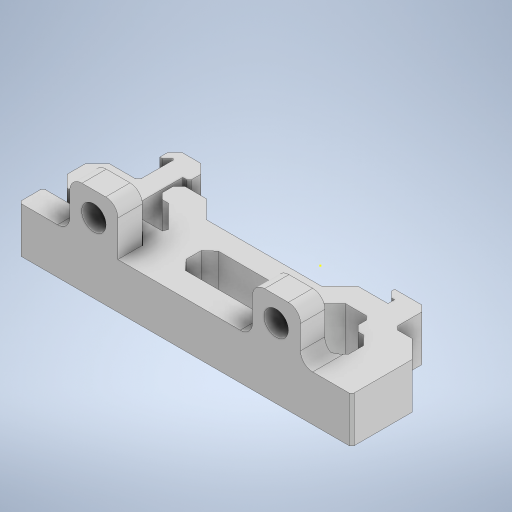
# Autodesk Inventor part: CO-1-01-lowPowerFuseMount
Saved by Autodesk Inventor 2024 (Build 280153000, 153)
## iProperties
Created: 2023-12-08
Part Number: CO-1-01-lowPowerFuseMount
Material: Generic
Document SubType Name: Modeling
Designer: t205b
Density: 1 g/cm^3
Appearance: Default
Author: t205b
Autodesk Inventor part; units mm, degrees
ref_plane "YZ Plane" through (0, 0, 0) normal (1, 0, 0) x (0, 1, 0)
ref_plane "XZ Plane" through (0, 0, 0) normal (0, 1, 0) x (-1, 0, 0)
ref_plane "XY Plane" through (0, 0, 0) normal (0, 0, 1) x (1, 0, 0)
sketch "Sketch1" plane through (0, 0, 0) normal (0, 1, 0) x (-1, 0, 0)
  point P0 (0, 0)
sketch "Sketch2" plane through (0, 0, 0) normal (0, 1, 0) x (-1, 0, 0)
  line L0 (-10.5015, 10.3489) -> (8.3899, 10.3489)
  line L1 (-25.4159, 10.3488) -> (-23.0295, 10.3488)
  line L2 (-26.8079, 11.7408) -> (-25.4159, 10.3488)
  line L3 (-28.3987, 13.3316) -> (-26.8079, 11.7408)
  line L4 (10.1121, 14.8658) -> (10.4033, 15.5686)
  line L5 (4.4127, 15.1552) -> (2.9213, 13.8428)
  line L6 (4.4127, 17.627) -> (2.9213, 19.2973)
  line L7 (25.8873, 23.2746) -> (-28.0034, 23.2746)
  line L8 (25.8893, 19.2989) -> (9.8813, 19.2989)
  line L9 (-22.433, 15.3341) -> (-20.9416, 13.8427)
  line L10 (25.8873, 23.2746) -> (26.2867, 22.8772)
  line L11 (26.2867, 22.8772) -> (26.2867, 19.6955)
  line L12 (26.2867, 19.6955) -> (25.8893, 19.2989)
  line L13 (9.8813, 19.2989) -> (11.8699, 17.3104)
  line L14 (11.8699, 17.3104) -> (24.2985, 17.3104)
  line L15 (24.2985, 17.3104) -> (26.287, 15.3218)
  line L16 (26.287, 15.3218) -> (26.287, 12.3389)
  line L17 (26.287, 12.3389) -> (24.2985, 10.3504)
  line L18 (24.2985, 10.3504) -> (20.0728, 10.3504)
  line L19 (20.0728, 10.3504) -> (19.5756, 9.8532)
  line L20 (19.5756, 9.8532) -> (19.5756, 4.6132)
  line L21 (19.5756, 4.6132) -> (19.8142, 4.3752)
  line L22 (19.8142, 4.3752) -> (20.719, 5.2815)
  line L23 (20.719, 5.2815) -> (21.1168, 5.2815)
  line L24 (21.1168, 5.2815) -> (21.1168, 3.9888)
  line L25 (21.1168, 3.9888) -> (19.9236, 2.7937)
  line L26 (19.9236, 2.7937) -> (16.8413, 2.7937)
  line L27 (16.8413, 2.7937) -> (15.3002, 4.3349)
  line L28 (15.3002, 5.9257) -> (15.3002, 4.3349)
  line L29 (15.6482, 6.2737) -> (16.3442, 6.2737)
  line L30 (10.1121, 14.8658) -> (13.8585, 11.1194)
  line L31 (13.8585, 11.1194) -> (14.8528, 11.1194)
  line L32 (14.8528, 11.1194) -> (15.847, 10.1252)
  line L33 (15.847, 10.1252) -> (15.847, 8.3603)
  line L34 (15.847, 8.3603) -> (14.8528, 7.366)
  line L35 (14.8528, 7.366) -> (11.3728, 7.366)
  line L36 (11.3728, 7.366) -> (8.3899, 10.3489)
  line L37 (-10.5015, 10.3489) -> (-13.4844, 7.366)
  line L38 (-13.4844, 7.366) -> (-18.4558, 7.366)
  line L39 (-18.4558, 7.366) -> (-18.4558, 6.2722)
  line L40 (-18.4558, 6.2722) -> (-17.9587, 6.2722)
  line L41 (-17.9587, 6.2722) -> (-16.9644, 5.2779)
  line L42 (-16.9644, 5.2779) -> (-16.9644, 4.7808)
  line L43 (-16.9644, 4.7808) -> (-21.4387, 4.7808)
  line L44 (-21.4387, 4.7808) -> (-22.433, 5.7751)
  line L45 (-22.433, 5.7751) -> (-22.433, 9.7522)
  line L46 (-22.433, 9.7522) -> (-23.0295, 10.3488)
  line L47 (-28.3987, 13.3316) -> (-28.3987, 22.8766)
  line L48 (-28.3987, 22.8766) -> (-28.0034, 23.2746)
  line L49 (-22.433, 15.3341) -> (-22.433, 17.8059)
  line L50 (-22.433, 17.8059) -> (-20.9416, 19.2973)
  line L51 (-20.9416, 19.2973) -> (2.9213, 19.2973)
  line L52 (4.4127, 17.627) -> (4.4127, 15.1552)
  line L53 (2.9213, 13.8428) -> (-11.9488, 13.8428)
  line L54 (-14.9316, 10.8599) -> (-18.4558, 10.8599)
  line L55 (-19.0524, 12.8485) -> (-20.0467, 13.8427)
  line L56 (-19.0524, 11.4565) -> (-19.0524, 12.8485)
  line L57 (-20.0467, 13.8427) -> (-20.9416, 13.8427)
  line L58 (-18.4558, 10.8599) -> (-19.0524, 11.4565)
  line L59 (-11.9488, 13.8428) -> (-14.9316, 10.8599)
  line L60 (19.3407, 12.8496) -> (19.3407, 14.8108)
  line L61 (19.3407, 14.8108) -> (23.2904, 14.8108)
  line L62 (23.2904, 14.8108) -> (23.7876, 14.3136)
  line L63 (23.7876, 14.3136) -> (23.7876, 13.3468)
  line L64 (23.7876, 13.3468) -> (23.2904, 12.8496)
  line L65 (23.2904, 12.8496) -> (19.3407, 12.8496)
  line L66 (15.6482, 6.2737) -> (15.3002, 5.9257)
  line L67 (16.3442, 15.0715) -> (16.3442, 6.2737)
  line L68 (15.847, 15.5686) -> (16.3442, 15.0715)
  line L69 (15.847, 15.5686) -> (10.4033, 15.5686)
  point P0 (0, 0)
  point P1 (-22.433, 16.57)
  dimension "d0" = 9.545
  dimension "d1" = 3.9771
  dimension "d2" = 4.4743
  dimension "d3" = 4.9714
  dimension "d4" = 3.5242
  dimension "d5" = 2.9829
  dimension "d6" = 0.9943
  dimension "d7" = 0.398
  dimension "d8" = 53.8907
  dimension "d9" = 2.4718
  dimension "d10" = 1.4914
  dimension "d11" = 1.4914
  dimension "d12" = 1.392
  dimension "d13" = 0.5966
  dimension "d14" = 23.8629
  dimension "d15" = 1.4914
  dimension "d16" = 2.4718
  dimension "d17" = 14.8701
  dimension "d18" = 2.9829
  dimension "d19" = 18.8914
  dimension "d20" = 2.9829
  dimension "d21" = 2.9829
  dimension "d22" = 3.48
  dimension "d23" = 3.7464
  dimension "d24" = 0.7028
  dimension "d25" = 5.4437
  dimension "d26" = 8.7978
  dimension "d27" = 0.4971
  dimension "d28" = 1.5909
  dimension "d29" = 0.348
  dimension "d30" = 0.696
  dimension "d31" = 1.5411
  dimension "d32" = 3.0823
  dimension "d33" = 1.1931
  dimension "d34" = 1.2927
  dimension "d35" = 0.3977
  dimension "d36" = 0.9048
  dimension "d37" = 0.2386
  dimension "d38" = 5.24
  dimension "d39" = 0.4971
  dimension "d40" = 4.2257
  dimension "d41" = 1.9886
  dimension "d42" = 2.9829
  dimension "d43" = 1.9886
  dimension "d44" = 12.4286
  dimension "d45" = 1.9886
  dimension "d46" = 16.008
  dimension "d47" = 0.3973
  dimension "d48" = 3.1817
  dimension "d49" = 2.9829
  dimension "d50" = 2.9829
  dimension "d51" = 2.9829
  dimension "d52" = 0.9943
  dimension "d53" = 0.9943
  dimension "d54" = 0.9943
  dimension "d55" = 3.7463
  dimension "d56" = 1.7649
  dimension "d57" = 0.9943
  dimension "d58" = 0.9943
  dimension "d59" = 0.4971
  dimension "d60" = 0.4971
  dimension "d61" = 0.4971
  dimension "d62" = 0.4971
  dimension "d63" = 0.4971
  constraints: 140 end point, 26 parallel, 17 perpendicular, 3 vertical, 1 horizontal, 1 midpoint
  measures "d0" distance of L47.end L3.start
  measures "d1" distance of L46.start L45.start
  measures "d2" distance of L44.start L43.start
  measures "d3" distance of L38.end L37.end
  measures "d4" distance of L54.start L54.end
  measures "d5" horizontal distance of L1.start L3.start
  measures "d6" horizontal distance of L45.start L44.start
  measures "d7" vertical distance of L7.end L47.end
  measures "d8" distance of L7.start L7.end
  measures "d9" distance of L9.start L49.end
  measures "d10" horizontal distance of L49.end L51.start
  measures "d11" horizontal distance of L9.start L57.end
  measures "d12" distance of L58.end L56.end
  measures "d13" vertical distance of L54.end L58.end
  measures "d14" distance of L51.start L6.end
  measures "d15" horizontal distance of L6.start L6.end
  measures "d16" distance of L6.start L5.start
  measures "d17" distance of L5.end L59.start
  measures "d18" horizontal distance of L59.start L54.start
  measures "d19" distance of L0.end L37.start
  measures "d20" horizontal distance of L37.end L37.start
  measures "d21" horizontal distance of L0.end L36.start
  measures "d22" distance of L36.start L35.start
  measures "d23" horizontal distance of L30.end L4.start
  measures "d24" vertical distance of L4.start L4.end
  measures "d25" distance of L4.end L68.start
  measures "d26" distance of L67.start L67.end
  measures "d27" horizontal distance of L68.start L67.start
  measures "d28" distance of L28.start L28.end
  measures "d29" horizontal distance of L28.start L29.start
  measures "d30" distance of L67.end L29.start
  measures "d31" horizontal distance of L28.end L26.end
  measures "d32" distance of L26.end L25.end
  measures "d33" horizontal distance of L25.end L24.end
  measures "d34" distance of L24.end L23.end
  measures "d35" distance of L23.end L23.start
  measures "d36" horizontal distance of L23.start L22.start
  measures "d37" horizontal distance of L22.start L20.end
  measures "d38" distance of L20.end L19.end
  measures "d39" horizontal distance of L19.end L19.start
  measures "d40" distance of L19.start L18.start
  measures "d41" horizontal distance of L16.end L18.start
  measures "d42" distance of L15.end L16.end
  measures "d43" horizontal distance of L15.start L15.end
  measures "d44" distance of L15.start L13.end
  measures "d45" horizontal distance of L13.start L13.end
  measures "d46" distance of L13.start L8.start
  measures "d47" horizontal distance of L8.start L12.start
  measures "d48" distance of L12.start L10.end
  measures "d49" horizontal distance of L37.end L37.start
  measures "d50" horizontal distance of L59.start L54.start
  measures "d51" horizontal distance of L0.end L36.start
  measures "d52" horizontal distance of L33.start L31.end
  measures "d53" horizontal distance of L33.start L31.end
  measures "d54" distance of L31.end L30.end
  measures "d55" vertical distance of L30.end L4.start
  measures "d56" distance of L33.end L33.start
  measures "d57" horizontal distance of L35.start L33.end
  measures "d58" horizontal distance of L35.start L33.end
  measures "d59" horizontal distance of L19.end L19.start
  measures "d60" horizontal distance of L63.end L65.start
  measures "d61" horizontal distance of L63.end L65.start
  measures "d62" horizontal distance of L61.end L62.end
  measures "d63" horizontal distance of L61.end L62.end
extrude "Extrusion1" add sketch "Sketch2" along normal blind 7.5
sketch "Sketch3" plane through (-25.8873, 0, 23.2746) normal (0, 0, 1) x (1, 0, 0)
  line L0 (0, 0) -> (53.8907, 0) projected
  line L1 (53.8907, 0) -> (53.8907, 7.5) projected
  line L2 (0, 7.5) -> (53.8907, 7.5) projected
  line L3 (0, 0) -> (0, 7.5) projected
  line L4 (7.9953, 7.5) -> (7.9953, 15.4)
  line L5 (7.9953, 15.4) -> (15.8953, 15.4)
  line L6 (15.8953, 15.4) -> (15.8953, 7.5)
  line L7 (37.9953, 7.5) -> (37.9953, 15.4)
  line L8 (37.9953, 15.4) -> (45.8953, 15.4)
  line L9 (45.8953, 15.4) -> (45.8953, 7.5)
  point P0 (25.8873, 0)
  dimension "d94" = 7.9
  dimension "d95" = 7.9
  dimension "d96" = 7.9
  dimension "d97" = 22.1
  dimension "d98" = 53.8907
  dimension "d99" = 7.9953
  constraints: 12 end point, 6 point on line, 3 perpendicular, 1 parallel, 1 vertical
  measures "d94" distance between parallel lines of L7 L9
  measures "d95" distance between parallel lines of L8 L2
  measures "d96" distance between parallel lines of L4 L6
  measures "d97" distance between parallel lines of L7 L6
  measures "d98" distance between parallel lines of L3 L1
  measures "d99" distance between parallel lines of L4 L3
extrude "Extrusion2" add sketch "Sketch3" against normal blind 4 contours L4 L5 L6 L2 | L2 L7 L8 L9
fillet "Fillet1" radius 2 7 edges at (-17.892, 15.4, 21.2746) (-17.892, 7.5, 21.2868) (-9.992, 15.4, 21.2746) (12.108, 15.4, 21.2746) (20.008, 15.4, 21.2746) (20.008, 7.5, 21.286) (12.108, 7.5, 21.286)
sketch "Sketch4" plane through (-25.8873, 0, 23.2746) normal (0, 0, 1) x (1, 0, 0)
  arc A0 (45.8953, 13.4) -> (43.8953, 15.4) centre (43.8953, 13.4) ccw projected
  line L0 (43.8953, 15.4) -> (39.9953, 15.4) projected
  arc A1 (39.9953, 15.4) -> (37.9953, 13.4) centre (39.9953, 13.4) ccw projected
  line L1 (37.9953, 13.4) -> (37.9953, 9.5) projected
  arc A2 (35.9953, 7.5) -> (37.9953, 9.5) centre (35.9953, 9.5) ccw projected
  line L2 (15.8953, 7.5) -> (35.9953, 7.5) projected
  line L3 (15.8953, 7.5) -> (15.8953, 13.4) projected
  arc A3 (15.8953, 13.4) -> (13.8953, 15.4) centre (13.8953, 13.4) ccw projected
  line L4 (13.8953, 15.4) -> (9.9953, 15.4) projected
  arc A4 (9.9953, 15.4) -> (7.9953, 13.4) centre (9.9953, 13.4) ccw projected
  line L5 (7.9953, 13.4) -> (7.9953, 9.5) projected
  arc A5 (5.9953, 7.5) -> (7.9953, 9.5) centre (5.9953, 9.5) ccw projected
  line L6 (0, 7.5) -> (5.9953, 7.5) projected
  line L7 (0, 0) -> (0, 7.5) projected
  line L8 (0, 0) -> (53.8907, 0) projected
  line L9 (53.8907, 0) -> (53.8907, 7.5) projected
  line L10 (47.8953, 7.5) -> (53.8907, 7.5) projected
  arc A6 (45.8953, 9.5) -> (47.8953, 7.5) centre (47.8953, 9.5) ccw projected
  line L11 (45.8953, 9.5) -> (45.8953, 13.4) projected
  point P0 (25.8873, 0)
  point P1 (11.9453, 11.45)
  point P2 (41.8953, 11.45)
  dimension "d112" = 3.95
  dimension "d113" = 3.95
  dimension "d116" = 29.95
  measures "d112" distance from line of point (11.945, 11.45) L4
  measures "d113" distance from line of L0 point (41.895, 11.45)
  measures "d116" distance of point (41.895, 11.45) point (11.945, 11.45)
hole "Hole1" at (-13.942, 11.45, 23.2746) at (16.008, 11.45, 23.2746) direction (0, 0, -1) diameter 4 end through all
equation "\"d95\" = d94"
equation "\"d96\" = d95"
equation "\"d99\" = -d94 + 0.5 * d98 - 0.5 * d97"
body "Solid1"
